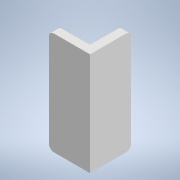
# Autodesk Inventor part: wheelguardbracket
Saved by Autodesk Inventor 2020.1 (Build 241239000, 239)
## iProperties
Created: 2019-12-09
Part Number: wheelguardbracket
Material: Generic
Document SubType Name: Modeling
Designer: tbloo
Density: 1 g/cm^3
Appearance: Default
Author: tbloo
Autodesk Inventor part; units mm, degrees
ref_plane "YZ Plane" through (0, 0, 0) normal (1, 0, 0) x (0, 1, 0)
ref_plane "XZ Plane" through (0, 0, 0) normal (0, 1, 0) x (-1, 0, 0)
ref_plane "XY Plane" through (0, 0, 0) normal (0, 0, 1) x (1, 0, 0)
sketch "Sketch1" plane through (0, 0, 0) normal (0, 1, 0) x (-1, 0, 0)
  line L0 (0, 0) -> (16, 0)
  line L1 (16, 0) -> (16, -3.2)
  line L2 (16, -3.2) -> (3.2, -3.2)
  line L3 (0, -3.2) -> (0, 0)
  line L4 (0, 0) -> (3.2, 0)
  line L5 (3.2, -3.2) -> (3.2, -16)
  line L6 (3.2, -16) -> (0, -16)
  line L7 (0, -16) -> (0, 0)
  dimension "d0" = 16
  dimension "d1" = 3.2
  dimension "d2" = 3.2
  dimension "d3" = 16
  constraints: 16 end point, 4 parallel, 2 horizontal, 2 perpendicular
  measures "d0" distance of L1.end L3.start
  measures "d1" distance of L0.end L1.end
  measures "d2" distance of L5.end L6.end
  measures "d3" distance of L4.end L5.end
extrude "Extrusion1" add sketch "Sketch1" along normal blind 40
fillet "Fillet1" radius 2 4 edges at (-1.6, 40, -16) (-16, 40, -1.6) (-1.6, 0, -16) (-16, 0, -1.6)
sketch "Sketch4" plane through (0, 0, 0) normal (1, 0, 0) x (0, 0, -1)
  circle A0 centre (9.6, 16) radius 1.85
  circle A1 centre (9.6, 32) radius 1.85
  point P0 (0, 0)
  constraints: 2 centre point, 4 other
sketch "Sketch5" plane through (0, 0, 0) normal (0, 0, 1) x (1, 0, 0)
  circle A0 centre (-9.6, 16) radius 1.85
  circle A1 centre (-9.6, 32) radius 1.85
  point P0 (0, 0)
  constraints: 2 centre point, 4 other
extrude "Extrusion4" cut sketch "Sketch4" against normal through all
extrude "Extrusion5" cut sketch "Sketch5" against normal through all
body "Solid1"
